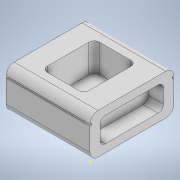
# Autodesk Inventor part: PassengerSectionGBR
Saved by Autodesk Inventor 2020.1 (Build 241239000, 239)
## iProperties
Created: 2020-02-27
Part Number: PassengerSectionGBR
Material: Generic
Document SubType Name: Modeling
Designer: super
Density: 1 g/cm^3
Appearance: Default
Author: super
Autodesk Inventor part; units mm, degrees
ref_plane "YZ Plane" through (0, 0, 0) normal (1, 0, 0) x (0, 1, 0)
ref_plane "XZ Plane" through (0, 0, 0) normal (0, 1, 0) x (-1, 0, 0)
ref_plane "XY Plane" through (0, 0, 0) normal (0, 0, 1) x (1, 0, 0)
sketch "Sketch1" plane through (0, 0, 0) normal (0, 1, 0) x (-1, 0, 0)
  point P0 (0, 0)
sketch "Sketch2" plane through (0, 0, 0) normal (0, 1, 0) x (-1, 0, 0)
  line L0 (0, 0) -> (80.518, 0)
  line L1 (80.518, 0) -> (80.518, -80.518)
  line L2 (80.518, -80.518) -> (0, -80.518)
  line L3 (0, -80.518) -> (0, 0)
  dimension "d0" = 80.518
  dimension "d1" = 80.518
  constraints: 8 end point, 2 parallel, 1 horizontal, 1 perpendicular
  measures "d0" distance of L1.end L2.end
  measures "d1" distance of L0.end L1.end
extrude "Extrusion1" add sketch "Sketch2" along normal blind 38.862
fillet "Fillet1" radius 7.62 4 edges at (-40.259, 0, 0) (-40.259, 38.862, 0) (-40.259, 0, -80.518) (-40.259, 38.862, -80.518)
sketch "Sketch3" plane through (0, 38.862, 0) normal (0, 1, 0) x (1, 0, 0)
  line L0 (-80.518, 80.518) -> (0, 80.518) projected
  line L1 (0, 7.62) -> (0, 72.898) projected
  line L2 (-20.828, 65.278) -> (-61.214, 65.278)
  line L3 (-61.214, 65.278) -> (-61.214, 14.986)
  line L4 (-61.214, 14.986) -> (-20.828, 14.986)
  line L5 (-20.828, 14.986) -> (-20.828, 65.278)
  point P0 (0, 0)
  dimension "d7" = 40.386
  dimension "d8" = 50.292
  constraints: 8 end point, 2 parallel, 1 horizontal, 1 perpendicular
  measures "d7" distance of L4.end L3.end
  measures "d8" distance of L3.end L2.end
extrude "Extrusion2" cut sketch "Sketch3" against normal blind 27.178
fillet "Fillet2" radius 5.08 4 edges at (-61.214, 25.273, -14.986) (-61.214, 25.273, -65.278) (-20.828, 25.273, -14.986) (-20.828, 25.273, -65.278)
sketch "Sketch4" plane through (0, 0, -7.62) normal (1, 0, 0) x (0, 0, -1)
  line L0 (72.898, 7.62) -> (72.898, 31.242) projected
  line L1 (62.992, 31.242) -> (2.032, 31.242)
  line L2 (2.032, 31.242) -> (2.032, 7.62)
  line L3 (2.032, 7.62) -> (62.992, 7.62)
  line L4 (62.992, 7.62) -> (62.992, 31.242)
  point P0 (-7.62, 0)
  dimension "d12" = 9.906
  dimension "d13" = 60.96
  dimension "d14" = 23.622
  constraints: 8 end point, 2 parallel, 1 horizontal, 1 perpendicular
  measures "d12" distance of L0.end L1.start
  measures "d13" distance of L3.end L2.end
  measures "d14" distance of L2.end L1.end
extrude "Extrusion3" cut sketch "Sketch4" against normal blind 14.478
fillet "Fillet3" radius 5.08 4 edges at (-7.239, 31.242, -9.652) (-7.239, 7.62, -9.652) (-7.239, 7.62, -70.612) (-7.239, 31.242, -70.612)
sketch "Sketch5" plane through (0, 31.242, -80.518) normal (0, 0, -1) x (-1, 0, 0)
  line L0 (0, 0) -> (0, -5.08) projected
  line L1 (0, 0) -> (0, -1.524)
  line L2 (0, -1.524) -> (80.518, -1.524)
  line L3 (80.518, -23.622) -> (80.518, 0) projected
  line L4 (80.518, 0) -> (0, 0) projected
  line L5 (80.518, 0) -> (0, 0)
  point P0 (0, -31.242)
  dimension "d18" = 1.524
  constraints: 6 end point, 2 point on line, 1 collinear, 1 perpendicular
  measures "d18" distance of L0.start L1.end
extrude "Extrusion4" cut sketch "Sketch5" against normal blind 1.524
sketch "Sketch6" plane through (-80.518, 31.242, 0) normal (0, 0, 1) x (1, 0, 0)
  line L0 (0, 0) -> (0, 7.62) projected
  line L1 (0, 0) -> (0, -1.524)
  line L2 (0, -23.622) -> (0, 0) projected
  line L3 (0, -1.524) -> (80.518, -1.524) projected
  line L4 (0, -1.524) -> (80.518, -1.524)
  line L5 (80.518, -5.08) -> (80.518, 0) projected
  line L6 (80.518, -1.524) -> (80.518, 0)
  line L7 (80.518, 0) -> (0, 0) projected
  line L8 (80.518, 0) -> (0, 0)
  point P0 (80.518, -31.242)
  dimension "d21" = 1.524
  constraints: 8 end point, 2 collinear, 1 perpendicular, 1 point on line
  measures "d21" distance of L0.start L1.end
extrude "Extrusion5" cut sketch "Sketch6" against normal blind 1.524
sketch "Sketch7" plane through (-80.518, 0, -72.898) normal (-1, 0, 0) x (0, 0, 1)
  arc A0 (72.898, 31.242) -> (65.278, 38.862) centre (65.278, 31.242) ccw projected
  line L0 (64.2238, 32.0041) -> (0.7238, 32.0041)
  line L1 (0.7238, 32.0041) -> (0.7238, 6.6041)
  line L2 (0.7238, 6.6041) -> (64.2238, 6.6041)
  line L3 (64.2238, 6.6041) -> (64.2238, 32.0041)
  point P0 (72.898, 0)
  dimension "d26" = 63.5
  dimension "d27" = 25.4
  constraints: 8 end point, 2 parallel, 1 horizontal, 1 perpendicular
  measures "d26" distance of L2.end L1.end
  measures "d27" distance of L1.end L0.end
extrude "Extrusion6" cut sketch "Sketch7" against normal blind 14.478
fillet "Fillet4" radius 5.08 4 edges at (-73.279, 32.0041, -72.1742) (-73.279, 6.6041, -72.1742) (-73.279, 6.6041, -8.6742) (-73.279, 32.0041, -8.6742)
body "Solid1"
